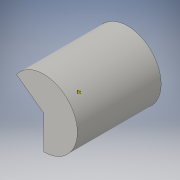
# Autodesk Inventor part: Part1
Saved by Autodesk Inventor 2016 (Build 200138000, 138)
## iProperties
Created: 2018-04-03
Part Number: Part1
Material: Generic
Document SubType Name: Modeling
Designer: Marek Kiejza
Density: 1 g/cm^3
Appearance: Default
Project: firstMK
Description: Part__1_Marek
Cost Center: Financial`
Catalog Web Link: www.Engineer.ie
Vendor: Client
Engineer: Pat Smith
Authority: Menagment
Stock Number: s00173510
Author: User_MK
Title: project1
Subject: item1
Revision Number: 56287
Autodesk Inventor part; units mm, degrees
ref_plane "YZ Plane" through (0, 0, 0) normal (1, 0, 0) x (0, 1, 0)
ref_plane "XZ Plane" through (0, 0, 0) normal (0, 1, 0) x (-1, 0, 0)
ref_plane "XY Plane" through (0, 0, 0) normal (0, 0, 1) x (1, 0, 0)
sketch "Sketch1" plane through (0, 0, 0) normal (1, 0, 0) x (0, 1, 0)
  line L0 (5.7135, 13.7519) -> (0.5374, 13.7519)
  line L1 (0.5374, 13.7519) -> (0.5374, 0.8757)
  line L2 (0.5374, 0.8757) -> (5.7135, 0.8757)
  line L3 (5.7135, 0.8757) -> (5.7135, 13.7519)
  point P0 (0, 0)
  constraints: 8 end point, 2 parallel, 1 horizontal, 1 perpendicular
revolve "Revolution1" add sketch "Sketch1" angle 234 about axis through (0, 5.7135, 0.8757) along (0, 0, 1)
body "Solid1"
